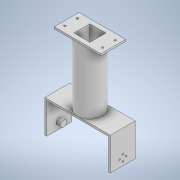
# Autodesk Inventor part: Tilt_Bracket_Output_2
Saved by Autodesk Inventor 2022 (Build 260153000, 153)
## iProperties
Created: 2022-02-11
Part Number: Tilt_Bracket_Output_2
Material: Generic
Document SubType Name: Modeling
Designer: Mlees
Density: 1 g/cm^3
Appearance: Default
Author: Mlees
Autodesk Inventor part; units mm, degrees
ref_plane "YZ Plane" through (0, 0, 0) normal (1, 0, 0) x (0, 1, 0)
ref_plane "XZ Plane" through (0, 0, 0) normal (0, 1, 0) x (-1, 0, 0)
ref_plane "XY Plane" through (0, 0, 0) normal (0, 0, 1) x (1, 0, 0)
sketch "Sketch1" plane through (0, 0, 0) normal (0, 0, 1) x (1, 0, 0)
  line L0 (0, 0) -> (0, 45)
  line L1 (0, 45) -> (98, 45)
  line L2 (98, 45) -> (98, 0)
  line L3 (98, 0) -> (101, 0)
  line L4 (101, 0) -> (101, 48)
  line L5 (101, 48) -> (-3, 48)
  line L6 (-3, 48) -> (-3, 0)
  line L7 (-3, 0) -> (0, 0)
  dimension "d0" = 45
  dimension "d1" = 98
  dimension "d2" = 3
  dimension "d3" = 48
  dimension "d4" = 104
  constraints: 16 end point, 6 perpendicular, 1 horizontal, 1 point on line, 1 vertical
  measures "d0" distance of L0.start L0.end
  measures "d1" distance of L0.end L1.end
  measures "d2" distance of L2.end L3.end
  measures "d3" distance of L3.end L4.end
  measures "d4" distance of L4.end L5.end
extrude "Extrusion1" add sketch "Sketch1" along normal blind 25.4
sketch "Sketch2" plane through (101, 0, 0) normal (1, 0, 0) x (0, 0, -1)
  line L0 (0, 0) -> (-25.4, 0) projected
  circle A0 centre (-12.7, 12) radius 1.125
  circle A1 centre (-17.7, 7) radius 1.125
  circle A2 centre (-12.7, 2) radius 1.125
  circle A3 centre (-7.7, 7) radius 1.125
  point P0 (-12.7, 7)
  dimension "d10" = 2.25
  dimension "d13" = 360
  constraints: 4 centre point, 9 other
  measures "d10" diameter of A0
extrude "Extrusion2" cut sketch "Sketch2" against normal up to surface (3 mm away)
sketch "Sketch3" plane through (98, 0, 0) normal (-1, 0, 0) x (0, 0, 1)
  circle A0 centre (12.7, 2) radius 1.125 projected
  circle A1 centre (12.7, 12) radius 1.125 projected
  circle A2 centre (12.7, 7) radius 8
  line L0 (12.7, 2) -> (12.7, 7)
  point P0 (0, 0)
  dimension "d21" = 16
  constraints: 2 end point, 1 centre point, 1 vertical
  measures "d21" diameter of A2
extrude "Extrusion3" cut sketch "Sketch3" against normal blind 1
sketch "Sketch4" plane through (98, 0, 0) normal (0, -1, 0) x (1, 0, 0)
  line L0 (0, 0) -> (0, 25.4) projected
  line L1 (3, 0) -> (3, 25.4) projected
  line L2 (0, 25.4) -> (3, 25.4)
  line L3 (3, 25.4) -> (3, 0)
  line L4 (3, 0) -> (0, 0)
  line L5 (0, 0) -> (0, 25.4)
  line L6 (-98, 0) -> (0, 0) projected
  line L7 (-101, 0) -> (-101, 25.4) projected
  line L8 (-98, 0) -> (-101, 0)
  line L9 (-101, 0) -> (-101, 25.4)
  line L10 (-101, 25.4) -> (-98, 25.4)
  line L11 (-98, 25.4) -> (-98, 0)
  point P0 (0, 12.7)
  point P1 (0, 12.7)
  constraints: 16 end point, 4 parallel, 2 horizontal, 2 perpendicular
extrude "Extrusion4" add sketch "Sketch4" along normal blind 4
sketch "Sketch5" plane through (98, 45, 0) normal (-1, 0, 0) x (0, 0, 1)
  arc A0 (16.573, -45) -> (8.827, -45) centre (12.7, -38) ccw projected
  circle A1 centre (12.7, -38) radius 8
  point P0 (0, -45)
  point P1 (8.827, -45)
  constraints: 1 centre point, 1 coincident
extrude "Extrusion5" cut sketch "Sketch5" against normal blind 1
sketch "Sketch6" plane through (0, 45, 25.4) normal (1, 0, 0) x (0, 0, -1)
  line L0 (25.4, -49) -> (0, -49) projected
  circle A0 centre (12.7, -38) radius 5
  point P0 (25.4, -45)
  point P1 (16.9, -49)
  point P2 (8.5, -49)
  dimension "d26" = 10
  constraints: 1 centre point
  measures "d26" diameter of A0
extrude "Extrusion6" add sketch "Sketch6" along normal blind 7
sketch "Sketch8" plane through (0, 0, 25.4) normal (0, 0, 1) x (1, 0, 0)
  line L0 (-3, -4) -> (0, -4) projected
  line L1 (-3, -4) -> (0, -4)
  line L2 (0, 45) -> (0, -4) projected
  line L3 (0, -4) -> (0, 45)
  line L4 (0, 45) -> (98, 45) projected
  line L5 (0, 45) -> (98, 45)
  line L6 (98, 45) -> (98, -4) projected
  line L7 (98, 45) -> (98, -4)
  line L8 (101, -4) -> (98, -4) projected
  line L9 (98, -4) -> (101, -4)
  line L10 (101, 48) -> (-3, 48) projected
  line L11 (101, -4) -> (101, 48)
  line L12 (101, 48) -> (-3, 48)
  line L13 (-3, 48) -> (-3, -4) projected
  line L14 (-3, 48) -> (-3, -4)
  point P0 (0, 0)
  constraints: 16 end point, 5 perpendicular, 2 collinear, 1 horizontal
extrude "Extrusion7" add sketch "Sketch8" along normal blind 7
sketch "Sketch9" plane through (0, 0, 0) normal (0, 0, -1) x (-1, 0, 0)
  line L0 (-98, -4) -> (-101, -4) projected
  line L1 (-101, 48) -> (-101, -4) projected
  line L2 (-101, -4) -> (-101, 48)
  line L3 (3, 48) -> (3, -4) projected
  line L4 (-101, 48) -> (3, 48)
  line L5 (3, 48) -> (3, -4)
  line L6 (3, -4) -> (0, -4) projected
  line L7 (3, -4) -> (0, -4)
  line L8 (0, 45) -> (0, -4) projected
  line L9 (0, -4) -> (0, 45)
  line L10 (-98, 45) -> (-98, -4) projected
  line L11 (0, 45) -> (-98, 45)
  line L12 (-98, 45) -> (-98, -4)
  line L13 (-98, -4) -> (-101, -4)
  point P0 (0, 0)
  constraints: 16 end point, 4 collinear, 4 perpendicular
extrude "Extrusion8" add sketch "Sketch9" along normal blind 7
sketch "Sketch10" plane through (-3, 48, 32.4) normal (0, 1, 0) x (1, 0, 0)
  line L0 (101, 39.4) -> (3, 39.4) projected
  line L1 (3, 0) -> (101, 0) projected
  circle A0 centre (52, 19.7) radius 19.7
  point P0 (3, 32.4)
  constraints: 1 centre point
extrude "Extrusion9" add sketch "Sketch10" along normal blind 101.6
sketch "Sketch11" plane through (49, 149.6, 12.7) normal (0, 1, 0) x (1, 0, 0)
  line L0 (-12.7, -12.7) -> (12.7, -12.7)
  line L1 (12.7, -12.7) -> (12.7, 12.7)
  line L2 (12.7, 12.7) -> (-12.7, 12.7)
  line L3 (-12.7, 12.7) -> (-12.7, -12.7)
  point P0 (-49, 12.7)
  dimension "d45" = 25.4
  dimension "d46" = 25.4
  constraints: 8 end point, 2 parallel, 1 horizontal, 1 perpendicular
  measures "d45" distance of L2.end L1.end
  measures "d46" distance of L1.end L0.end
extrude "Extrusion10" cut sketch "Sketch11" against normal through all
sketch "Sketch12" plane through (49, 149.6, 12.7) normal (0, 1, 0) x (1, 0, 0)
  line L0 (49, -19.7) -> (52, -19.7) projected
  line L1 (-52, 19.7) -> (-52, -19.7) projected
  line L2 (52, -19.7) -> (-52, -19.7)
  line L3 (-49, 19.7) -> (-52, 19.7) projected
  line L4 (-52, -19.7) -> (-52, 19.7)
  line L5 (52, -19.7) -> (52, 19.7) projected
  line L6 (-52, 19.7) -> (52, 19.7)
  line L7 (52, 19.7) -> (52, -19.7)
  line L8 (12.7, -12.7) -> (12.7, 12.7) projected
  line L9 (12.7, -12.7) -> (12.7, 12.7)
  line L10 (12.7, 12.7) -> (-12.7, 12.7) projected
  line L11 (12.7, 12.7) -> (-12.7, 12.7)
  line L12 (-12.7, -12.7) -> (-12.7, 12.7) projected
  line L13 (-12.7, 12.7) -> (-12.7, -12.7)
  line L14 (-12.7, -12.7) -> (12.7, -12.7) projected
  line L15 (-12.7, -12.7) -> (12.7, -12.7)
  point P0 (-49, 12.7)
  constraints: 16 end point, 4 collinear, 4 perpendicular
extrude "Extrusion16" add sketch "Sketch12" along normal blind 3
sketch "Sketch17" plane through (49, 149.6, 12.7) normal (0, -1, 0) x (1, 0, 0)
  line L0 (-52, -19.7) -> (-52, 19.7) projected
  arc A0 (0, 19.7) -> (0, -19.7) centre (0, 0) ccw projected
  circle A1 centre (-30, 10) radius 1.5
  circle A2 centre (-30, -10) radius 1.5
  circle A3 centre (30, -10) radius 1.5
  circle A4 centre (30, 10) radius 1.5
  point P0 (-49, -12.7)
  constraints: 4 centre point
extrude "Extrusion17" cut sketch "Sketch17" against normal through all
sketch "Sketch18" plane through (-3, 149.6, -7) normal (-1, 0, 0) x (0, 0, 1)
  line L0 (0, 0) -> (0, 3) projected
  line L1 (39.4, 0) -> (39.4, 3) projected
  line L2 (0, 3) -> (39.4, 3)
  line L3 (39.4, 3) -> (39.4, 0)
  line L4 (39.4, 0) -> (0, 0)
  line L5 (0, 0) -> (0, 3)
  point P0 (7, -149.6)
  constraints: 8 end point, 2 parallel, 1 horizontal, 1 perpendicular
extrude "Extrusion18" cut sketch "Sketch18" against normal blind 15
sketch "Sketch19" plane through (101, 149.6, 32.4) normal (1, 0, 0) x (0, 0, -1)
  line L0 (0, 0) -> (0, 3) projected
  line L1 (0, 3) -> (39.4, 3) projected
  line L2 (0, 0) -> (39.4, 0)
  line L3 (39.4, 0) -> (39.4, 3)
  line L4 (39.4, 3) -> (0, 3)
  line L5 (0, 3) -> (0, 0)
  point P0 (32.4, -149.6)
  constraints: 8 end point, 2 parallel, 1 horizontal, 1 perpendicular
extrude "Extrusion19" cut sketch "Sketch19" against normal blind 15
body "Solid1"
